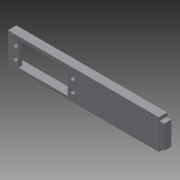
# Autodesk Inventor part: servo_holder
Saved by Autodesk Inventor 2015 SP2 (Build 190223200, 223)
## iProperties
Created: 2016-08-31
Part Number: servo_holder
Material: Generic
Document SubType Name: Modeling
Designer: jm799
Density: 1 g/cm^3
Appearance: Default
Author: jm799
Autodesk Inventor part; units mm, degrees
ref_plane "YZ Plane" through (0, 0, 0) normal (1, 0, 0) x (0, 1, 0)
ref_plane "XZ Plane" through (0, 0, 0) normal (0, 1, 0) x (-1, 0, 0)
ref_plane "XY Plane" through (0, 0, 0) normal (0, 0, 1) x (1, 0, 0)
sketch "Sketch2" plane through (0, 0, 0) normal (0, 1, 0) x (-1, 0, 0)
  line L0 (0, 0) -> (60, 0)
  line L1 (60, 0) -> (60, 25)
  line L2 (60, 25) -> (0, 25)
  line L3 (0, 25) -> (0, 0)
  dimension "d2" = 25
  dimension "d3" = 60
  constraints: 8 end point, 2 parallel, 1 horizontal, 1 perpendicular
  measures "d2" distance of L2.end L0.start
  measures "d3" distance of L1.end L2.end
extrude "Extrusion1" add sketch "Sketch2" along normal blind 3
sketch "Sketch4" plane through (0, 3, 0) normal (0, 1, 0) x (1, 0, 0)
  line L0 (-60, 0) -> (-60, -25) construction
  line L1 (-60, -12.5) -> (-56, -12.5) construction
  circle A0 centre (-54.0543, -17.5142) radius 2
  circle A1 centre (-54.0543, -7.5142) radius 2
  line L2 (-60, -25) -> (0, -25) projected
  line L3 (0, 0) -> (-60, 0) projected
  circle A2 centre (-6.3738, -17.5142) radius 2
  circle A3 centre (-6.3738, -7.5142) radius 2
  line L4 (-50, -21) -> (-9.77, -21)
  line L5 (-9.77, -21) -> (-9.77, -4)
  line L6 (-9.77, -4) -> (-50, -4)
  line L7 (-50, -4) -> (-50, -21)
  line L8 (-54.0543, -17.5142) -> (-51.0543, -17.5142)
  line L9 (-54.0543, -7.5142) -> (-51.0543, -7.5142)
  line L10 (-6.3738, -17.5142) -> (-9.3738, -17.5142)
  line L11 (-6.3738, -7.5142) -> (-9.3738, -7.5142)
  dimension "d8" = 4
  dimension "d9" = 4
  dimension "d11" = 40.23
  dimension "d12" = 3
  dimension "d13" = 3
  dimension "d14" = 3
  dimension "d15" = 3
  constraints: 18 end point, 5 horizontal, 4 centre point, 2 parallel, 1 coincident, 1 midpoint, 1 perpendicular
  measures "d8" diameter of A0
  measures "d9" diameter of A1
  measures "d11" distance of L6.end L5.end
  measures "d12" distance of L8.start L8.end
  measures "d13" distance of L9.start L9.end
  measures "d14" distance of L10.start L10.end
  measures "d15" distance of L11.start L11.end
hole "Hole1" at (-54.0543, 3, 17.5142) at (-54.0543, 3, 7.5142) at (-6.3738, 3, 17.5142) at (-6.3738, 3, 7.5142) direction (0, -1, 0) diameter 4 depth 8 tip angle 118
sketch "Sketch8" plane through (0, 3, 0) normal (0, 1, 0) x (1, 0, 0)
  circle A0 centre (-54.0543, -17.5142) radius 2 projected
  line L0 (-54.0543, -17.5142) -> (-51.0543, -17.5142)
  circle A1 centre (-54.0543, -7.5142) radius 2 projected
  line L1 (-54.0543, -7.5142) -> (-51.0543, -7.5142)
  circle A2 centre (-6.3738, -17.5142) radius 2 projected
  line L2 (-6.3738, -17.5142) -> (-9.3738, -17.5142)
  circle A3 centre (-6.3738, -7.5142) radius 2 projected
  line L3 (-6.3738, -7.5142) -> (-9.3738, -7.5142)
  line L4 (-51.1048, -22.3867) -> (-10.1048, -22.3867)
  line L5 (-10.1048, -22.3867) -> (-10.1048, -2.3867)
  line L6 (-10.1048, -2.3867) -> (-51.1048, -2.3867)
  line L7 (-51.1048, -2.3867) -> (-51.1048, -22.3867)
  point P0 (0, 0)
  dimension "d23" = 3
  dimension "d24" = 3
  dimension "d25" = 3
  dimension "d26" = 3
  dimension "d27" = 20
  dimension "d30" = 41
  constraints: 16 end point, 5 horizontal, 2 parallel, 1 perpendicular
  measures "d23" distance of L0.start L0.end
  measures "d24" distance of L1.start L1.end
  measures "d25" distance of L2.start L2.end
  measures "d26" distance of L3.start L3.end
  measures "d27" distance of L4.end L5.end
  measures "d30" distance of L5.end L6.end
extrude "Extrusion2" cut sketch "Sketch8" against normal blind 3 contours L7 L6 L5 L4
sketch "Sketch10" plane through (0, 3, 0) normal (0, 1, 0) x (1, 0, 0)
  line L0 (0, -25) -> (0, 0) projected
  line L1 (-60, -25) -> (0, -25)
  line L2 (0, -25) -> (0, -22.3867)
  line L3 (0, -22.3867) -> (-60, -22.3867)
  line L4 (-60, -22.3867) -> (-60, -25)
  line L5 (-60, 0) -> (0, 0)
  line L6 (0, 0) -> (0, -2.3796)
  line L7 (0, -2.3796) -> (-60, -2.3796)
  line L8 (-60, -2.3796) -> (-60, 0)
  constraints: 16 end point, 4 parallel, 2 horizontal, 2 perpendicular, 2 point on line
extrude "Extrusion3" add sketch "Sketch10" along normal blind 4 and the other way blind 3
sketch "Sketch11" plane through (0, 0, 0) normal (0, -1, 0) x (1, 0, 0)
  line L0 (0, 0) -> (66, 0)
  line L1 (0, 25) -> (66, 25)
  line L2 (66, 0) -> (66, 25)
  line L3 (0, 0) -> (0, 25)
  line L4 (0, 25) -> (0, 0) projected
  dimension "d39" = 66
  constraints: 8 end point, 2 horizontal, 1 collinear, 1 vertical
  measures "d39" distance of L0.start L0.end
extrude "Extrusion4" add sketch "Sketch11" against normal blind 7
sketch "Sketch12" plane through (66, 0, 25) normal (1, 0, 0) x (0, 0, -1)
  line L0 (0, 0) -> (0, 7) construction
  line L1 (0, 0) -> (0, 7) construction
  line L2 (0, 3.5) -> (25, 3.5) construction
  line L3 (25, 0) -> (25, 7) construction
  line L4 (2.6133, 0) -> (22.6133, 0) construction
  line L5 (12.6133, 0) -> (12.6169, 7) construction
  line L6 (22.6204, 7) -> (2.6133, 7) construction
  line L7 (2.8651, 0.55) -> (22.3651, 0.55)
  line L8 (22.3651, 0.55) -> (22.3651, 6.45)
  line L9 (22.3651, 6.45) -> (2.8651, 6.45)
  line L10 (2.8651, 6.45) -> (2.8651, 0.55)
  line L11 (12.6151, 0.55) -> (12.6151, 6.45) construction
  line L12 (2.8651, 3.5) -> (22.3651, 3.5) construction
  point P0 (12.6151, 3.5)
  dimension "d42" = 19.5
  dimension "d43" = 5.9
  constraints: 18 end point, 10 midpoint, 3 equal length, 1 horizontal, 1 perpendicular
  measures "d42" distance of L9.end L8.end
  measures "d43" distance of L8.end L7.end
extrude "Extrusion5" add sketch "Sketch12" along normal blind 4
body "Solid1"
